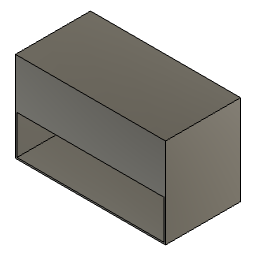
Cabinet (Autodesk Fusion 360 design; units mm, degrees)
Autodesk Fusion 360 part; units mm, degrees
sketch "Sketch1" plane through (0, 0, 0) normal (0, 0, 1) x (1, 0, 0)
  line L0 (-50, -25) -> (50, -25)
  line L1 (50, -25) -> (50, 25)
  line L2 (50, 25) -> (-50, 25)
  line L3 (-50, 25) -> (-50, -25)
  constraint horizontal L0
  constraint vertical L1
  constraint horizontal L2
  constraint vertical L3
extrude "Extrude1" add sketch "Sketch1" along normal blind 1
sketch "Sketch2" plane through (0, 0, 1) normal (0, 0, 1) x (-1, 0, 0)
  line L0 (50, -25) -> (50, 25)
  line L1 (50, 25) -> (-50, 25)
  line L2 (-50, 25) -> (-50, -25)
  line L3 (-50, -25) -> (50, -25)
  line L4 (49, 24) -> (-49, 24)
  line L5 (-49, 24) -> (-49, -24)
  line L6 (-49, -24) -> (49, -24)
  line L7 (49, -24) -> (49, 24)
  line L8 (49, 24) -> (49, 25)
  line L9 (-49, 24) -> (-49, 25)
  dimension "d3" = -1
  constraint coincident L1 L8.end
  constraint perpendicular L1 L8
  constraint coincident L1 L9.end
  constraint perpendicular L1 L9
extrude "Extrude2" add sketch "Sketch2" along normal blind 59 contours L0 L1 L2 L3 L5 L6 L7 L8 L9
sketch "Sketch3" plane through (0, 0, 60) normal (0, 0, 1) x (-1, 0, 0)
  line L0 (-49, -24) -> (-49, 25)
  line L1 (-49, 25) -> (-50, 25)
  line L2 (-50, 25) -> (-50, -25)
  line L3 (-50, -25) -> (50, -25)
  line L4 (50, -25) -> (50, 25)
  line L5 (50, 25) -> (49, 25)
  line L6 (49, 25) -> (49, -24)
  line L7 (49, -24) -> (-49, -24)
  line L8 (50, -25) -> (-50, -25)
  line L9 (-50, -25) -> (-50, 25)
  line L10 (-50, 25) -> (50, 25)
  line L11 (50, 25) -> (50, -25)
  constraint horizontal L8
  constraint vertical L9
  constraint horizontal L10
  constraint vertical L11
  constraint coincident L1.end L2.start
  constraint coincident L3.end L4.start
extrude "Extrude3" add sketch "Sketch3" against normal blind 1 contours L0 L6 L7 L10
sketch "Sketch4" plane through (0, 0, 59) normal (0, 0, -1) x (1, 0, 0)
  line L0 (-49, -24) -> (49, -24)
  line L1 (49, -24) -> (49, 25)
  line L2 (49, 25) -> (-49, 25)
  line L3 (-49, 25) -> (-49, -24)
  line L4 (-49, 25) -> (-49, 24)
  line L5 (-49, 24) -> (49, 24)
  dimension "d8" = 1
  constraint coincident L2.end L3.start
  constraint perpendicular L2 L4
  constraint coincident L1 L5.end
  constraint perpendicular L1 L5
  measures "d8" distance of L2.end L4.end
extrude "Extrude4" add sketch "Sketch4" along normal blind 32 contours L1 L2 L3 L4 L5
